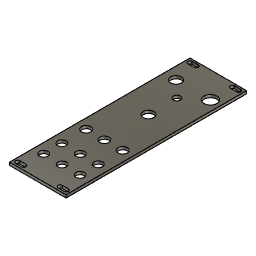
ujoveFIXED v5 (Autodesk Fusion 360 design; units mm, degrees)
Autodesk Fusion 360 part; units mm, degrees
sketch "Sketch1" plane through (0, 0, 0) normal (0, 0, 1) x (1, 0, 0)
  line L0 (0, 0) -> (40.3, 0)
  line L1 (40.3, 0) -> (40.3, 128.54)
  line L2 (40.3, 128.54) -> (0, 128.54)
  line L3 (0, 128.54) -> (0, 0)
  line L4 (0, 0) -> (0, 3) construction
  line L5 (0, 3) -> (40.3, 3) construction
  line L6 (0, 0) -> (0, 17.3) construction
  line L7 (0, 17.3) -> (40.3, 17.3) construction
  line L8 (0, 17.3) -> (0, 30.3) construction
  line L9 (0, 30.3) -> (0, 47.6) construction
  line L10 (0, 47.6) -> (40.3, 47.6) construction
  line L11 (0, 30.3) -> (40.3, 30.3) construction
  line L12 (0, 47.6) -> (0, 78.9) construction
  line L13 (0, 78.9) -> (40.3, 78.9) construction
  line L14 (0, 78.9) -> (0, 99.2) construction
  line L15 (0, 99.2) -> (40.3, 99.2) construction
  line L16 (0, 128.54) -> (0, 110.04) construction
  line L17 (0, 110.04) -> (40.3, 110.04) construction
  line L18 (0, 0) -> (7, 0) construction
  line L19 (7, 0) -> (7, 47.6) construction
  line L20 (7, 0) -> (20, 0) construction
  line L21 (20, 0) -> (20, 47.6) construction
  line L22 (20, 0) -> (33, 0) construction
  line L23 (33, 0) -> (33, 47.6) construction
  circle A0 centre (7, 30.3) radius 3
  circle A1 centre (7, 17.3) radius 3
  circle A2 centre (20.15, 30.3) radius 3
  circle A3 centre (20.15, 17.3) radius 3
  circle A4 centre (33, 30.3) radius 3
  circle A5 centre (33, 17.3) radius 3
  circle A6 centre (7, 47.6) radius 3.3
  circle A7 centre (20, 47.6) radius 3.3
  circle A8 centre (33, 47.6) radius 3.3
  line L24 (0, 78.9) -> (20.15, 78.9) construction
  circle A9 centre (20.15, 78.9) radius 3.8
  line L25 (0, 99.2) -> (20.15, 99.2) construction
  circle A10 centre (20.15, 99.2) radius 2.5
  line L26 (0, 110.04) -> (0.6568, 110.04) construction
  line L27 (0, 110.04) -> (8.6, 110.04) construction
  line L28 (8.6, 110.04) -> (33.1, 110.04) construction
  circle A11 centre (8.6, 110.04) radius 3.8
  circle A12 centre (33.1, 110.04) radius 4.65
  line L29 (0, 3) -> (5, 3) construction
  line L30 (5, 3) -> (5, 4.5) construction
  line L31 (5, 3) -> (5, 1.5) construction
  line L32 (5, 1.5) -> (7.225, 1.5)
  line L33 (5, 1.5) -> (2.775, 1.5)
  line L34 (5, 4.5) -> (7.225, 4.5)
  line L35 (5, 4.5) -> (2.775, 4.5)
  line L36 (2.775, 3) -> (1.275, 3)
  arc A13 (2.775, 4.5) -> (2.775, 1.5) centre (2.775, 3) ccw
  line L37 (7.225, 3) -> (8.725, 3)
  arc A14 (7.225, 1.5) -> (7.225, 4.5) centre (7.225, 3) ccw
  arc A15 (2.775, 4.5) -> (2.775, 1.5) centre (2.775, 3) ccw
  line L38 (5, 4.5) -> (2.775, 4.5)
  line L39 (5, 4.5) -> (7.225, 4.5)
  arc A16 (7.225, 1.5) -> (7.225, 4.5) centre (7.225, 3) ccw
  line L40 (5, 1.5) -> (7.225, 1.5)
  line L41 (5, 1.5) -> (2.775, 1.5)
  line L42 (40.3, 0) -> (35.3, 0) construction
  line L43 (35.3, 0) -> (35.3, 3) construction
  arc A17 (33.075, 4.5) -> (33.075, 1.5) centre (33.075, 3) ccw
  line L44 (35.3, 4.5) -> (33.075, 4.5)
  line L45 (35.3, 4.5) -> (37.525, 4.5)
  line L46 (35.3, 1.5) -> (33.075, 1.5)
  line L47 (35.3, 1.5) -> (37.525, 1.5)
  arc A18 (37.525, 1.5) -> (37.525, 4.5) centre (37.525, 3) ccw
  line L48 (0, 128.54) -> (0, 125.74) construction
  line L49 (0, 125.74) -> (40.3, 125.74) construction
  line L50 (0, 125.74) -> (5, 125.74) construction
  line L51 (40.3, 125.74) -> (35.3, 125.74) construction
  arc A19 (2.775, 127.24) -> (2.775, 124.24) centre (2.775, 125.74) ccw
  line L52 (5, 127.24) -> (2.775, 127.24)
  line L53 (5, 127.24) -> (7.225, 127.24)
  line L54 (5, 124.24) -> (2.775, 124.24)
  line L55 (5, 124.24) -> (7.225, 124.24)
  arc A20 (7.225, 124.24) -> (7.225, 127.24) centre (7.225, 125.74) ccw
  arc A21 (33.075, 127.24) -> (33.075, 124.24) centre (33.075, 125.74) ccw
  line L56 (35.3, 127.24) -> (33.075, 127.24)
  line L57 (35.3, 127.24) -> (37.525, 127.24)
  line L58 (35.3, 124.24) -> (33.075, 124.24)
  line L59 (35.3, 124.24) -> (37.525, 124.24)
  arc A22 (37.525, 124.24) -> (37.525, 127.24) centre (37.525, 125.74) ccw
  dimension "d1" = 40.3
  dimension "d2" = 128.54
  dimension "d3" = 3
  dimension "d5" = 17.3
  dimension "d6" = 13
  dimension "d7" = 17.3
  dimension "d8" = 31.3
  dimension "d9" = 20.3
  dimension "d10" = 18.5
  dimension "d11" = 7
  dimension "d12" = 13
  dimension "d13" = 13
  dimension "d14" = 6
  dimension "d15" = 6
  dimension "d16" = 6
  dimension "d17" = 6
  dimension "d18" = 6
  dimension "d19" = 6
  dimension "d20" = 6.6
  dimension "d21" = 6.6
  dimension "d22" = 6.6
  dimension "d23" = 7.6
  dimension "d24" = 5
  dimension "d25" = 8.6
  dimension "d26" = 24.5
  dimension "d27" = 7.6
  dimension "d28" = 9.3
  dimension "d29" = 5
  dimension "d30" = 1.5
  dimension "d31" = 1.5
  dimension "d32" = 2.225
  dimension "d33" = 2.225
  dimension "d35" = 2.225
  dimension "d36" = 2.225
  dimension "d37" = 1.5
  dimension "d38" = 1.5
  dimension "d39" = 2.225
  dimension "d40" = 2.225
  dimension "d41" = 2.225
  dimension "d42" = 2.225
  dimension "d43" = 5
  dimension "d44" = 2.225
  dimension "d45" = 2.225
  dimension "d46" = 2.225
  dimension "d47" = 2.225
  dimension "d48" = 2.225
  dimension "d49" = 2.8
  dimension "d50" = 5
  dimension "d51" = 5
  dimension "d52" = 2.225
  dimension "d53" = 2.225
  dimension "d54" = 2.225
  dimension "d56" = 2.225
  dimension "d57" = 2.225
  dimension "d58" = 2.225
  dimension "d59" = 2.225
  dimension "d61" = 2.225
  constraint horizontal L0
  constraint vertical L1
  constraint horizontal L2
  constraint vertical L3
  constraint coincident L0.start L3.end
  constraint perpendicular L0 L4
  constraint coincident L1 L5.end
  constraint perpendicular L1 L5
  constraint perpendicular L5 L6
  constraint coincident L1 L7.end
  constraint perpendicular L1 L7
  constraint perpendicular L7 L8
  constraint parallel L3 L9
  constraint coincident L1 L10.end
  constraint perpendicular L1 L10
  constraint coincident L1 L11.end
  constraint perpendicular L1 L11
  constraint perpendicular L10 L12
  constraint coincident L1 L13.end
  constraint perpendicular L1 L13
  constraint perpendicular L13 L14
  constraint coincident L1 L15.end
  constraint perpendicular L1 L15
  constraint perpendicular L2 L16
  constraint coincident L1 L17.end
  constraint perpendicular L1 L17
  constraint perpendicular L6 L18
  constraint coincident L10 L19.end
  constraint perpendicular L10 L19
  constraint perpendicular L19 L20
  constraint vertical L21
  constraint coincident L10 L21.end
  constraint perpendicular L21 L22
  constraint coincident L10 L23.end
  constraint perpendicular L10 L23
  constraint coincident L11 A0.centre
  constraint coincident L19 A0.centre
  constraint coincident L19 A1.centre
  constraint coincident L7 A1.centre
  constraint midpoint L11 A2.centre
  constraint midpoint L7 A3.centre
  constraint coincident L23 A4.centre
  constraint coincident L11 A4.centre
  constraint coincident L7 A5.centre
  constraint coincident L23 A5.centre
  constraint coincident L19.end A6.centre
  constraint coincident L21.end A7.centre
  constraint coincident L23.end A8.centre
  constraint midpoint L13 L24.end
  constraint coincident L24.end A9.centre
  constraint midpoint L15 L25.end
  constraint coincident L25.end A10.centre
  constraint coincident L17 L26.end
  constraint perpendicular L16 L26
  constraint perpendicular L3 L27
  constraint parallel L17 L28
  constraint coincident L27.end L28.start
  constraint coincident L28.end A12.centre
  constraint perpendicular L6 L29
  constraint perpendicular L29 L30
  constraint perpendicular L29 L31
  constraint perpendicular L31 L32
  constraint perpendicular L31 L33
  constraint perpendicular L30 L34
  constraint perpendicular L30 L35
  constraint coincident L36.end A13
  constraint coincident L5 L37.start
  constraint parallel L5 L37
  constraint coincident L37.end A14
  constraint perpendicular L1 L42
  constraint coincident L5 L43.end
  constraint perpendicular L5 L43
  constraint perpendicular L2 L48
  constraint coincident L1 L49.end
  constraint perpendicular L1 L49
  constraint perpendicular L16 L50
  constraint perpendicular L1 L51
  measures "d1" distance of L0.start L0.end
  measures "d2" distance of L0.start L2.end
  measures "d3" distance of L0.start L4.end
  measures "d5" distance of L0.start L6.end
  measures "d6" distance of L6.end L8.end
  measures "d7" distance of L8.end L9.end
  measures "d8" distance of L9.end L12.end
  measures "d9" distance of L12.end L14.end
  measures "d10" distance of L2.end L16.end
  measures "d11" distance of L0.start L18.end
  measures "d12" distance of L18.end L20.end
  measures "d13" distance of L20.end L22.end
  measures "d14" diameter of A0
  measures "d15" diameter of A1
  measures "d16" diameter of A2
  measures "d17" diameter of A3
  measures "d18" diameter of A4
  measures "d19" diameter of A5
  measures "d20" diameter of A6
  measures "d21" diameter of A7 L8
  measures "d22" diameter of A8
  measures "d23" diameter of A9
  measures "d24" diameter of A10
  measures "d25" distance of L16.end L27.end
  measures "d26" distance of L27.end L28.end
  measures "d27" diameter of A11
  measures "d28" diameter of A12
  measures "d29" distance of L4.end L29.end
  measures "d30" distance of L29.end L30.end
  measures "d31" distance of L29.end L31.end
  measures "d32" distance of L31.end L32.end
  measures "d33" distance of L31.end L33.end
  measures "d35" distance of L30.end L34.end
  measures "d36" distance of L30.end L35.end
  measures "d37" distance of L36.start L36.end
  measures "d38" distance of L37.start L37.end
  measures "d39" distance of L31.end L32.end
  measures "d40" distance of L31.end L33.end
  measures "d41" distance of L30.end L34.end
  measures "d42" distance of L35.end L30.end
  measures "d43" distance of L0.end L42.end
  measures "d44" distance of L46.start L47.end
  measures "d45" distance of L46.start A17.end
  measures "d46" distance of L44.start L45.end
  measures "d47" distance of L45.end L44.start
  measures "d48" distance of A17.start L44.start
  measures "d49" distance of L2.end L48.end
  measures "d50" distance of L48.end L50.end
  measures "d51" distance of L49.end L51.end
  measures "d52" distance of L54.start L55.end
  measures "d53" distance of L54.start A19.end
  measures "d54" distance of L52.start L53.end
  measures "d56" distance of A19.start L52.start
  measures "d57" distance of L58.start L59.end
  measures "d58" distance of L58.start A21.end
  measures "d59" distance of L56.start L57.end
  measures "d61" distance of A21.start L56.start
extrude "Extrude1" add sketch "Sketch1" along normal blind 2
equation "d32 = ( 4.45 / 2 ) * 1 mm"
equation "d33 = ( 4.45 / 2 ) * 1 mm"
equation "d35 = ( 4.45 / 2 ) * 1 mm"
equation "d36 = ( 4.45 / 2 ) * 1 mm"
equation "d39 = ( 4.45 / 2 ) * 1 mm"
equation "d40 = ( 4.45 / 2 ) * 1 mm"
equation "d41 = ( 4.45 / 2 ) * 1 mm"
equation "d42 = ( 4.45 / 2 ) * 1 mm"
equation "d44 = ( 4.45 / 2 ) * 1 mm"
equation "d45 = ( 4.45 / 2 ) * 1 mm"
equation "d46 = ( 4.45 / 2 ) * 1 mm"
equation "d47 = ( 4.45 / 2 ) * 1 mm"
equation "d48 = ( 4.45 / 2 ) * 1 mm"
equation "d52 = ( 4.45 / 2 ) * 1 mm"
equation "d53 = ( 4.45 / 2 ) * 1 mm"
equation "d54 = ( 4.45 / 2 ) * 1 mm"
equation "d56 = ( 4.45 / 2 ) * 1 mm"
equation "d57 = ( 4.45 / 2 ) * 1 mm"
equation "d58 = ( 4.45 / 2 ) * 1 mm"
equation "d59 = ( 4.45 / 2 ) * 1 mm"
equation "d61 = ( 4.45 / 2 ) * 1 mm"
